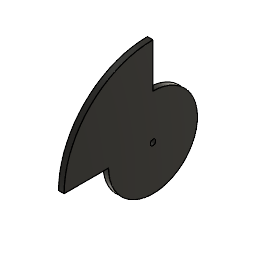
Obturator (Autodesk Fusion 360 design; units mm, degrees)
part number: 2026-06-02-09-22-29-568
Autodesk Fusion 360 part; units mm, degrees
note: some values were not read from the file. Set by a fixed rule: which sketch regions a step uses.
sketch "Obturator" plane through (0, 0, 0) normal (1, 0, 0) x (0, 1, 0)
  circle A0 centre (0, 0) radius 80
  line L0 (85, 85) -> (-85, 85)
  line L1 (-85, 85) -> (-85, -85)
  line L2 (-85, -85) -> (85, -85)
  line L3 (85, -85) -> (85, 85)
  line L4 (85, 85) -> (-85, -85) construction
  line L5 (-85, 85) -> (85, -85) construction
  line L6 (-55, 55) -> (-30.5, 55)
  line L7 (-30.5, 55) -> (-30.5, 36)
  line L8 (-30.5, 36) -> (-55, 36)
  line L9 (-55, 36) -> (-55, 55)
  circle A1 centre (0, 0) radius 40
  line L10 (0, 0) -> (0, 80)
  line L11 (0, 0) -> (-80, 0)
  circle A2 centre (0, 0) radius 2.5
  dimension "d1" = 160
  dimension "d2" = 170
  dimension "d3" = 170
  dimension "d4" = 24.5
  dimension "d5" = 19
  dimension "d6" = 30
  dimension "d7" = 30
  dimension "d8" = 80
  dimension "d9" = 5
  constraint coincident A0.centre A1.centre
  constraint horizontal L0
  constraint perpendicular L0 L1
  constraint parallel L0 L2
  constraint parallel L1 L3
  constraint coincident L4 A0.centre
  constraint coincident L5 A0.centre
  constraint horizontal L6
  constraint vertical L7
  constraint horizontal L8
  constraint vertical L9
  constraint coincident A0 L10.end
  constraint perpendicular L0 L10
  constraint coincident A0 L11.end
  constraint perpendicular L10 L11
  constraint concentric A1 A2
  measures "d1" diameter of A0
  measures "d2" distance of L1.end L2.end
  measures "d3" distance of L0.end L1.end
  measures "d4" distance of L6.start L6.end
  measures "d5" distance of L6.start L8.end
  measures "d6" distance of L0 L6
  measures "d7" distance of L1 L9
  measures "d8" diameter of A1
  measures "d9" diameter of A2
extrude "Extrude1" add sketch "Obturator" along normal blind 5 contours A0 A1 L10 L11 | A1 L10 L11 A2 | A1 L10 L11 A2 | L6 L7 L8 L9 picked at (-15.8593, 57.9262)
named bodies: "Obturator"
